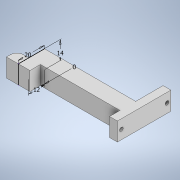
# Autodesk Inventor part: AdaptadorSensorAnycubic
Saved by Autodesk Inventor 2020.3 (Build 243373000, 373)
## iProperties
Created: 2020-09-07
Part Number: AdaptadorSensorAnycubic
Material: Generic
Document SubType Name: Modeling
Designer: mifer
Density: 1 g/cm^3
Appearance: Default
Author: mifer
## iProperties of the stored document _3DPrint.ipt
Created: 2020-09-09
Part Number: _3DPrint
Material: Generic
Document SubType Name: Modeling
Designer: mifer
Density: 1 g/cm^3
Appearance: Default
Author: mifer
Autodesk Inventor part; units mm, degrees
ref_plane "YZ Plane" through (0, 0, 0) normal (1, 0, 0) x (0, 1, 0)
ref_plane "XZ Plane" through (0, 0, 0) normal (0, 1, 0) x (-1, 0, 0)
ref_plane "XY Plane" through (0, 0, 0) normal (0, 0, 1) x (1, 0, 0)
sketch "Sketch1" plane through (0, 0, 0) normal (1, 0, 0) x (0, 1, 0)
  line L0 (0, 0) -> (14, 0)
  line L1 (14, 0) -> (14, -20)
  line L2 (14, -20) -> (0, -20)
  line L3 (0, -20) -> (0, 0)
  line L4 (14, -20) -> (0, -20)
  line L5 (0, -20) -> (0, -20)
  line L6 (0, -20) -> (14, -20)
  line L7 (14, -20) -> (14, -20)
  line L8 (0, 0) -> (0, -8)
  line L9 (0, -8) -> (14, -8)
  line L10 (14, -8) -> (14, 0)
  point P0 (14, -8)
  dimension "d12" = 14
  dimension "d13" = 20
  dimension "d14" = 12
  dimension "d15" = 0
  constraints: 22 end point, 5 equal length, 3 point on line, 2 horizontal, 2 perpendicular
  measures "d12" distance of L1.end L2.end
  measures "d13" distance of L0.end L1.end
  measures "d14" distance between parallel lines of L4 L9
  measures "d15" distance between parallel lines of L2 L4
extrude "Extrusion6" add sketch "Sketch1" along normal blind 70 contours L9 L1 L2 L3
extrude "Extrusion7" add sketch "Sketch1" against normal mid plane 18 contours L0 L1 L9 L3
fillet "Fillet1" radius 5 1 edges at (-9, 7, -8)
sketch "Sketch6" plane through (70, 0, 0) normal (1, 0, 0) x (0, 0, -1)
  line L0 (8, 14) -> (0, 14) projected
  line L1 (0, 14) -> (41, 14)
  line L2 (41, 14) -> (41, 0)
  line L3 (41, 0) -> (0, 0)
  line L4 (0, 0) -> (0, 14)
  circle A0 centre (38, 7) radius 1.4
  circle A1 centre (3, 7) radius 1.4
  line L5 (8, 14) -> (8, 0) projected
  dimension "d21" = 41
  dimension "d22" = 2.8
  dimension "d23" = 3
  dimension "d24" = 2.8
  dimension "d25" = 35
  dimension "d26" = 5
  constraints: 8 end point, 2 centre point, 2 parallel, 1 horizontal, 1 perpendicular
  measures "d21" distance of L2.end L3.end
  measures "d22" diameter of A0
  measures "d23" distance from line of L2 A0.centre
  measures "d24" diameter of A1
  measures "d25" distance of A0.centre A1.centre
  measures "d26" distance from line of L5 A1.centre
extrude "Extrusion8" add sketch "Sketch6" along normal blind 6
body "Solid2"
